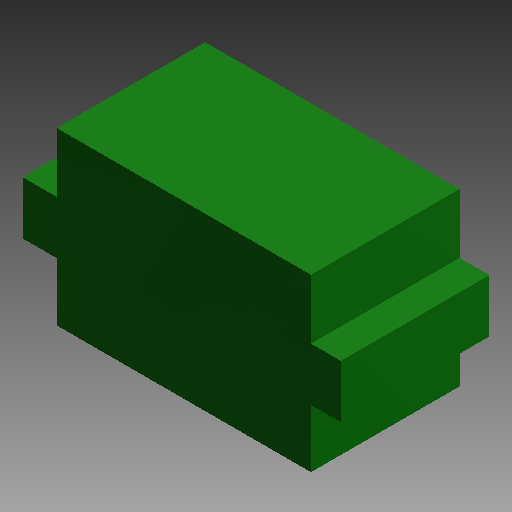
# Autodesk Inventor part: 1N4148WT
Saved by Autodesk Inventor 2018.2 (Build 222227000, 227)
## iProperties
Part Number: 1N4148WT
Material: Generic
Document SubType Name: Modeling
Designer: autocad
Appearance: SOD523, 1N4148WT
Author: autocad
Autodesk Inventor part; units mm, degrees
ref_plane "YZ Plane" through (0, 0, 0) normal (1, 0, 0) x (0, 1, 0)
ref_plane "XZ Plane" through (0, 0, 0) normal (0, 1, 0) x (-1, 0, 0)
ref_plane "XY Plane" through (0, 0, 0) normal (0, 0, 1) x (1, 0, 0)
sketch "SOD523, 1N4148WT_101" plane through (0, 0, 0) normal (0, 0, 1) x (1, 0, 0)
  line L0 (0.6091, 0.125) -> (0.75, 0.125)
  line L1 (0.75, 0.125) -> (0.75, -0.125)
  line L2 (0.75, -0.125) -> (0.6091, -0.125)
  line L3 (0.6091, -0.125) -> (0.6091, -0.3995)
  line L4 (0.6091, -0.3995) -> (-0.5895, -0.3995)
  line L5 (-0.5895, -0.3995) -> (-0.5895, -0.125)
  line L6 (-0.5895, -0.125) -> (-0.75, -0.125)
  line L7 (-0.75, -0.125) -> (-0.75, 0.125)
  line L8 (-0.75, 0.125) -> (-0.5895, 0.125)
  line L9 (-0.5895, 0.125) -> (-0.5895, 0.4059)
  line L10 (-0.5895, 0.4059) -> (0.6091, 0.4059)
  line L11 (0.6091, 0.4059) -> (0.6091, 0.125)
  constraints: 24 end point
extrude "Extrusion1" add sketch "SOD523, 1N4148WT_101" along normal blind 0.7
body "Solid1"
